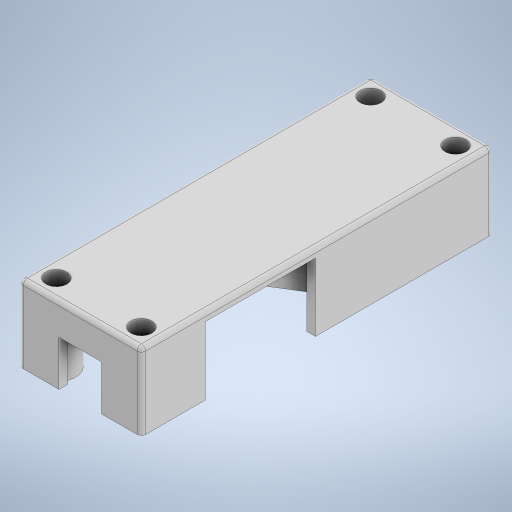
# Autodesk Inventor part: CaseTop
Saved by Autodesk Inventor 2023 (Build 270158000, 158)
## iProperties
Created: 2022-10-21
Part Number: CaseTop
Material: Generic
Document SubType Name: Modeling
Designer: Intern
Density: 1 g/cm^3
Appearance: Default
Author: Intern
Autodesk Inventor part; units mm, degrees
ref_plane "YZ Plane" through (0, 0, 0) normal (1, 0, 0) x (0, 1, 0)
ref_plane "XZ Plane" through (0, 0, 0) normal (0, 1, 0) x (-1, 0, 0)
ref_plane "XY Plane" through (0, 0, 0) normal (0, 0, 1) x (1, 0, 0)
sketch "Sketch1" plane through (0, 0, 0) normal (0, 1, 0) x (-1, 0, 0)
  line L0 (-4.1759, -63.8889) -> (-35.6719, -63.8889)
  line L1 (-35.6719, -63.8889) -> (-35.6719, 36.1871)
  line L2 (-35.6719, 36.1871) -> (-4.1759, 36.1871)
  line L3 (-4.1759, 36.1871) -> (-4.1759, -63.8889)
  line L4 (-1.6359, -66.4289) -> (-38.2119, -66.4289)
  line L5 (-38.2119, -66.4289) -> (-38.2119, 38.7271)
  line L6 (-38.2119, 38.7271) -> (-1.6359, 38.7271)
  line L7 (-1.6359, 38.7271) -> (-1.6359, -66.4289)
  point P0 (0, 0)
  dimension "d0" = 100.076
  dimension "d1" = 31.496
  dimension "d2" = 2.54
  dimension "d3" = 2.54
  dimension "d4" = 2.54
  dimension "d5" = 2.54
  constraints: 16 end point, 4 parallel, 2 horizontal, 2 perpendicular
  measures "d0" distance of L0.end L1.end
  measures "d1" distance of L1.end L2.end
  measures "d2" distance between parallel lines of L5 L1
  measures "d3" distance between parallel lines of L3 L7
  measures "d4" distance between parallel lines of L0 L4
  measures "d5" distance between parallel lines of L2 L6
extrude "Extrusion1" add sketch "Sketch1" along normal blind 22.86 contours L0 L1 L2 L3 | L4 L5 L6 L7
extrude "Extrusion2" cut sketch "Sketch1" along normal blind 20.32 contours L0 L1 L2 L3
sketch "Sketch2" plane through (0, 0, 0) normal (0, -1, 0) x (1, 0, 0)
  line L0 (35.6719, 36.1871) -> (35.6719, -63.8889) projected
  line L1 (38.2119, 38.7271) -> (38.2119, -66.4289) projected
  line L2 (38.2119, 19.6771) -> (35.6719, 19.6771)
  line L3 (38.2119, -13.3429) -> (35.6719, -13.3429)
  line L4 (4.1759, 36.1871) -> (35.6719, 36.1871) projected
  point P0 (0, 0)
  point P1 (36.9419, 19.6771)
  point P2 (36.9419, -13.3429)
  dimension "d10" = 16.51
  dimension "d11" = 33.02
  constraints: 4 end point, 4 point on line, 2 midpoint, 1 horizontal, 1 perpendicular
  measures "d10" distance from line of L4 point (36.942, 19.677)
  measures "d11" distance of point (36.942, 19.677) point (36.942, -13.343)
extrude "Extrusion3" cut sketch "Sketch2" against normal blind 20.32
sketch "Sketch3" plane through (1.6359, 0, 38.7271) normal (0, 0, 1) x (1, 0, 0)
  line L0 (11.938, 0) -> (24.638, 0)
  line L1 (24.638, 0) -> (24.638, 13.5128)
  line L2 (24.638, 13.5128) -> (11.938, 13.5128)
  line L3 (11.938, 13.5128) -> (11.938, 0)
  line L4 (0, 0) -> (0, 22.86) projected
  line L5 (36.576, 0) -> (36.576, 22.86) projected
  line L6 (36.576, 22.86) -> (0, 22.86) projected
  line L7 (18.288, 22.86) -> (18.288, 0)
  point P0 (-1.6359, 0)
  dimension "d16" = 13.5128
  dimension "d17" = 12.7
  dimension "d18" = 12.7
  constraints: 10 end point, 2 midpoint, 2 parallel, 2 perpendicular, 1 horizontal
  measures "d16" distance between parallel lines of L0 L2
  measures "d17" distance of L1.end L2.end
  measures "d18" diameter of L3 L7
extrude "Extrusion4" cut sketch "Sketch3" against normal blind 2.54
sketch "Sketch4" plane through (1.6359, 0, -66.4289) normal (-1, 0, 0) x (0, 0, 1)
  line L0 (12.192, 0) -> (51.3334, 0)
  line L1 (51.3334, 0) -> (51.3334, 12.7)
  line L2 (51.3334, 12.7) -> (12.192, 12.7)
  line L3 (12.192, 12.7) -> (12.192, 0)
  line L4 (0, 0) -> (0, 22.86) projected
  point P0 (66.4289, 0)
  point P1 (31.7627, 0)
  dimension "d21" = 12.192
  dimension "d22" = 12.7
  dimension "d23" = 39.1414
  constraints: 8 end point, 2 parallel, 1 horizontal, 1 midpoint, 1 perpendicular
  measures "d21" distance between parallel lines of L4 L3
  measures "d22" distance from line of point (31.763, 0) L2
  measures "d23" distance of L1.end L2.end
extrude "Extrusion5" cut sketch "Sketch4" against normal blind 2.54
sketch "Sketch5" plane through (0, 22.86, 0) normal (0, 1, 0) x (1, 0, 0)
  circle A0 centre (32.6239, -33.1391) radius 1.4732
  line L0 (38.2119, -38.7271) -> (38.2119, 66.4289) projected
  line L1 (1.6359, -38.7271) -> (38.2119, -38.7271) projected
  line L2 (1.6359, 66.4289) -> (1.6359, -38.7271) projected
  line L3 (1.6359, 13.8509) -> (38.2119, 13.8509)
  line L4 (19.9239, 66.4289) -> (19.9239, -38.7271)
  circle A1 centre (7.2239, -33.1391) radius 1.4732
  circle A2 centre (32.6239, 60.8409) radius 1.4732
  circle A3 centre (7.2239, 60.8409) radius 1.4732
  circle A4 centre (32.6239, -33.1391) radius 3.175
  line L5 (38.2119, -31.941) -> (38.2119, -34.3372)
  line L6 (31.4257, -38.7271) -> (33.822, -38.7271)
  arc A5 (38.2119, -31.941) -> (31.4257, -38.7271) centre (32.6239, -33.1391) ccw
  line L7 (38.2119, -34.3372) -> (38.2119, -38.7271)
  line L8 (38.2119, -38.7271) -> (33.822, -38.7271)
  line L9 (38.2119, -38.7271) -> (1.6359, -38.7271)
  circle A6 centre (7.2239, -33.1391) radius 3.175
  line L10 (1.6359, -31.941) -> (1.6359, -34.3372)
  arc A7 (8.422, -38.7271) -> (1.6359, -31.941) centre (7.2239, -33.1391) ccw
  line L11 (1.6359, -34.3372) -> (1.6359, -38.7271)
  line L12 (38.2119, 66.4289) -> (38.2119, -38.7271)
  line L13 (1.6359, -38.7271) -> (1.6359, 66.4289)
  circle A8 centre (32.6239, 60.8409) radius 3.175
  arc A9 (31.4257, 66.4289) -> (38.2119, 59.6428) centre (32.6239, 60.8409) ccw
  circle A10 centre (7.2239, 60.8409) radius 3.175
  arc A11 (1.6359, 59.6428) -> (8.422, 66.4289) centre (7.2239, 60.8409) ccw
  line L14 (38.2119, 66.4289) -> (1.6359, 66.4289)
  point P0 (0, 0)
  point P1 (1.6359, 59.6428)
  point P2 (38.2119, 59.6428)
  point P3 (8.422, -38.7271)
  point P4 (1.6359, -31.941)
  dimension "d27" = 2.9464
  dimension "d28" = 5.588
  dimension "d29" = 5.588
  dimension "d30" = 6.35
  constraints: 24 end point, 24 symmetric about line, 12 centre point, 8 point on circle, 7 point on line, 5 coincident, 3 midpoint, 2 collinear, 9 other
  measures "d27" diameter of A0
  measures "d28" distance from line of L0 A0.centre
  measures "d29" distance from line of L1 A0.centre
  measures "d30" diameter of A4
extrude "Extrusion6" add sketch "Sketch5" against normal up to surface (22.86 mm away) contours A0 | L1 A5 L0 | A9 L14 L0 | L1 L2 A7 | L2 L14 A11 | A1 | A2 | A3 | A4 | A6 | A8 | A10
extrude "Extrusion7" cut sketch "Sketch5" against normal blind 20.32 contours A0 | A1 | A2 | A3 | A4 | A6 | A8 | A10
extrude "Extrusion8" cut sketch "Sketch5" against normal blind 22.86 contours A0 | A1 | A2 | A3
fillet "Fillet2" radius 3.175 2 edges at (2.9059, 12.7, -54.2369) (2.9059, 12.7, -15.0955)
fillet "Fillet3" radius 1.27 8 edges at (38.2119, 22.86, -13.8509) (38.2119, 11.43, 38.7271) (19.9239, 22.86, 38.7271) (1.6359, 22.86, -13.8509) (38.2119, 11.43, -66.4289) (19.9239, 22.86, -66.4289) (1.6359, 11.43, 38.7271) (1.6359, 11.43, -66.4289)
sketch "Sketch8" plane through (0, 0, 0) normal (0, -1, 0) x (1, 0, 0)
  line L0 (1.6359, -15.0955) -> (4.1759, -15.0955) projected
  line L1 (4.1759, -15.0955) -> (17.1299, -15.0955)
  line L2 (17.1299, -15.0955) -> (17.1299, -54.5295)
  line L3 (17.1299, -54.5295) -> (4.1759, -54.5295)
  line L4 (4.1759, -54.5295) -> (4.1759, -15.0955)
  line L5 (35.6719, -13.3429) -> (35.6719, -56.0065) projected
  line L6 (35.6719, -13.3429) -> (24.7499, -13.3429)
  line L7 (24.7499, -13.3429) -> (24.7499, 19.5815)
  line L8 (24.7499, 19.5815) -> (35.6719, 19.5815)
  line L9 (35.6719, 19.5815) -> (35.6719, -13.3429)
  line L10 (4.1759, -4.9355) -> (35.6719, -24.2565)
  line L11 (4.1759, -4.9355) -> (4.1759, -2.3955)
  line L12 (2.9059, 37.4571) -> (2.9059, -65.1589) projected
  line L13 (35.6719, -24.2565) -> (35.6719, -21.7165)
  line L14 (4.1759, -2.3955) -> (35.6719, -21.7165)
  point P0 (0, 0)
  point P1 (24.7499, 3.1193)
  dimension "d44" = 10.922
  dimension "d45" = 12.954
  dimension "d46" = 2.54
  dimension "d47" = 2.54
  dimension "d48" = 31.75
  dimension "d49" = 10.16
  constraints: 24 end point, 6 parallel, 3 point on line, 2 horizontal, 2 perpendicular, 1 midpoint
  measures "d44" distance from line of L9 point (24.75, 3.119)
  measures "d45" distance between parallel lines of L4 L2
  measures "d46" distance of L10.end L13.end
  measures "d47" distance of L10.start L11.end
  measures "d48" distance of L5.end L10.end
  measures "d49" distance of L10.start L0.end
extrude "Extrusion11" add sketch "Sketch8" against normal blind 20.32 contours L5 L10 L11 L14
extrude "Extrusion12" cut sketch "Sketch8" against normal blind 5.08 contours L5 L10 L11 L14
fillet "Fillet4" radius 1.27 18 edges at (4.1759, 12.7, -2.3955) (4.1759, 20.32, 12.9546) (19.9239, 20.32, -12.056) (4.1759, 5.08, -3.6655) (19.9239, 20.32, -14.596) (35.6719, 12.7, -24.2565) (35.6719, 5.08, -22.9865) (35.6719, 20.32, -40.1315) (35.6719, 20.32, 23.9909) (28.5827, 20.32, 29.098) (19.9239, 20.32, 36.1871) (19.9239, 20.32, -63.8889) (28.5827, 20.32, -56.7998) (11.265, 20.32, -56.7998) (4.1759, 20.32, -30.471) (11.265, 20.32, 29.098) (4.1759, 12.7, -4.9355) (35.6719, 12.7, -21.7165)
body "Solid1"
